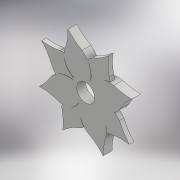
# Autodesk Inventor part: Hombro
Saved by Autodesk Inventor 2017 (Build 210142000, 142)
## iProperties
Created: 2018-06-14
Part Number: Hombro
Material: Generic
Document SubType Name: Modeling
Designer: Carolina Lema
Density: 1 g/cm^3
Appearance: Default
Author: Carolina Lema
Autodesk Inventor part; units mm, degrees
ref_plane "YZ Plane" through (0, 0, 0) normal (1, 0, 0) x (0, 1, 0)
ref_plane "XZ Plane" through (0, 0, 0) normal (0, 1, 0) x (-1, 0, 0)
ref_plane "XY Plane" through (0, 0, 0) normal (0, 0, 1) x (1, 0, 0)
sketch "Sketch1" plane through (0, 0, 0) normal (0, 1, 0) x (-1, 0, 0)
  circle A0 centre (0, 0) radius 3.1567
  arc A1 (0.8045, 7.8482) -> (-1.096, 2.9604) centre (3.8775, 3.84) ccw
  arc A2 (0.8045, 7.8482) -> (3.9995, 10.3658) centre (-5.1655, 18.7108) ccw
  arc A3 (3.9995, 10.3658) -> (4.6274, 6.3833) centre (14.1317, 9.9224) ccw
  arc A4 (2.723, 1.597) -> (4.6274, 6.3833) centre (0.993, 5.0574) ccw
  arc A5 (-2.811, -1.4364) -> (-4.581, -6.3031) centre (0.3797, -5.3521) ccw
  arc A6 (-3.9197, -10.3658) -> (-4.581, -6.3031) centre (-16.3145, -10.2983) ccw
  arc A7 (-0.7514, -7.7504) -> (-3.9197, -10.3658) centre (3.9871, -16.7173) ccw
  arc A8 (-0.7514, -7.7504) -> (1.0381, -2.9812) centre (-2.4622, -4.3882) ccw
  arc A9 (-4.581, 6.3031) -> (-3.9197, 10.3658) centre (-16.3145, 10.2983) ccw
  arc A10 (-3.9197, 10.3658) -> (-0.7514, 7.7504) centre (3.9871, 16.7173) ccw
  arc A11 (0.0827, -7.173) -> (0.8045, -7.8482) centre (3.8775, -3.84) ccw
  arc A12 (3.9995, -10.4433) -> (0.8045, -7.8482) centre (-5.3042, -18.6335) ccw
  arc A13 (4.6274, -6.3833) -> (3.9995, -10.4433) centre (14.1284, -9.9311) ccw
  arc A14 (4.6274, -6.3833) -> (4.8845, -4.8845) centre (1.1142, -5.0091) ccw
  arc A15 (-6.3833, -4.6274) -> (-4.6482, -4.8692) centre (-5.0091, -1.1142) ccw
  arc A16 (-1.4365, 2.8109) -> (-6.3031, 4.581) centre (-5.3521, -0.3794) ccw
  arc A17 (-7.7504, 0.7514) -> (-2.9812, -1.038) centre (-4.3883, 2.4621) ccw
  arc A18 (-6.3833, -4.6274) -> (-10.4433, -3.9995) centre (-9.9311, -14.1284) ccw
  arc A19 (-10.4433, -3.9995) -> (-7.8482, -0.8045) centre (-18.6335, 5.3042) ccw
  arc A20 (-7.7504, 0.7514) -> (-10.3658, 3.9197) centre (-16.7173, -3.9871) ccw
  arc A21 (-10.3658, 3.9197) -> (-6.3031, 4.581) centre (-10.2983, 16.3145) ccw
  arc A22 (-7.173, -0.0827) -> (-7.8482, -0.8045) centre (-3.84, -3.8775) ccw
  circle A23 centre (0, 0) radius 3.1567
  arc A24 (1.597, -2.723) -> (6.3833, -4.6274) centre (5.0091, -1.1142) ccw
  arc A25 (7.8482, -0.8045) -> (10.4433, -3.9995) centre (18.6335, 5.3042) ccw
  arc A26 (10.4433, -3.9995) -> (6.3833, -4.6274) centre (9.9311, -14.1284) ccw
  arc A27 (7.8482, -0.8045) -> (2.9604, 1.096) centre (3.84, -3.8775) ccw
  arc A28 (10.3658, 3.9197) -> (7.7544, 0.7514) centre (16.7241, -3.9816) ccw
  arc A29 (6.2595, 4.581) -> (10.3658, 3.9197) centre (10.2556, 16.3142) ccw
  arc A30 (-4.581, 6.3031) -> (-4.6176, 4.6176) centre (0.3794, 5.3521) ccw
  arc A31 (0.0827, 7.173) -> (-0.7514, 7.7504) centre (-2.4621, 4.3883) ccw
  arc A32 (6.2595, 4.581) -> (4.8322, 4.581) centre (5.5459, -0.4191) ccw
  arc A33 (7.173, -0.0827) -> (7.7544, 0.7514) centre (4.3971, 2.4718) ccw
  point P0 (0, 0)
  constraints: 82 point on circle, 34 centre point
extrude "Extrusion1" add sketch "Sketch1" along normal blind 2 contours A0 | A0 A27 A25 A26 A24 | A0 A1 A2 A3 A4 | A8 A7 A6 A5 A0 | A0 A17 A20 A21 A16
sketch "Sketch2" plane through (0, 0, 0) normal (0, -1, 0) x (1, 0, 0)
  arc A0 (-6.3002, -4.5761) -> (-10.3587, -3.9384) centre (-9.8712, -14.0685) ccw
  arc A1 (-10.3587, -3.9384) -> (-7.7558, -0.7497) centre (-18.5261, 5.3853) ccw
  arc A2 (-7.6963, 1.7106) -> (-6.727, 0.2513) centre (-4.1552, 3.0112) ccw
  arc A3 (-7.6963, 1.7106) -> (-9.9181, 5.1662) centre (-17.1611, -1.9329) ccw
  arc A4 (1.6813, 7.6084) -> (0.3953, 6.5184) centre (4.2581, 3.2645) ccw
  arc A5 (5.4246, 4.6938) -> (5.3039, 5.7011) centre (1.6527, 4.7526) ccw
  arc A6 (5.1612, 9.8069) -> (5.3039, 5.7011) centre (15.1582, 8.099) ccw
  arc A7 (1.6813, 7.6084) -> (5.1612, 9.8069) centre (-3.1073, 19.0411) ccw
  circle A8 centre (0, 0) radius 3.1567
  arc A9 (-2.939, 1.152) -> (-7.7558, -0.7497) centre (-3.7548, -3.8328) ccw
  arc A10 (-3.9384, 10.3587) -> (-0.7497, 7.7558) centre (5.3853, 18.5261) ccw
  arc A11 (1.1518, 2.9391) -> (-0.7497, 7.7558) centre (-3.8325, 3.7551) ccw
  arc A12 (-4.5761, 6.3002) -> (-3.9384, 10.3587) centre (-14.0685, 9.8712) ccw
  arc A13 (-4.8177, 5.3149) -> (-5.8057, 5.3418) centre (-5.4487, 0.3038) ccw
  arc A14 (-9.9181, 5.1662) -> (-5.8057, 5.3418) centre (-8.3835, 17.4659) ccw
  arc A15 (-4.5761, 6.3002) -> (-2.7536, 1.5435) centre (-1.0663, 4.9175) ccw
  circle A16 centre (0, 0) radius 3.1567
  arc A17 (7.5795, -1.6487) -> (9.8069, -5.1612) centre (19.0125, 3.1391) ccw
  arc A18 (9.8069, -5.1612) -> (5.7037, -5.3068) centre (8.1076, -15.1596) ccw
  arc A19 (7.5795, -1.6487) -> (6.6332, -0.5802) centre (3.3633, -4.4295) ccw
  arc A20 (10.4117, 3.8786) -> (7.8466, 0.7681) centre (16.7974, -4.0005) ccw
  arc A21 (4.6938, -5.4246) -> (5.7037, -5.3068) centre (4.7657, -1.6529) ccw
  arc A22 (6.4086, 4.6012) -> (10.4117, 3.8786) centre (10.5823, 16.2725) ccw
  arc A23 (3.0009, -0.9796) -> (7.8466, 0.7681) centre (4.4443, 2.6098) ccw
  arc A24 (6.4086, 4.6012) -> (1.4895, 2.7832) centre (5.4455, -0.3568) ccw
  arc A25 (4.6012, -6.4086) -> (2.7832, -1.4895) centre (-0.3568, -5.4455) ccw
  arc A26 (-1.7106, -7.6963) -> (-5.1662, -9.9181) centre (1.9329, -17.1611) ccw
  arc A27 (-1.7106, -7.6963) -> (-0.4181, -6.895) centre (-3.0112, -4.1552) ccw
  arc A28 (-5.1662, -9.9181) -> (-5.3418, -5.8057) centre (-17.4659, -8.3835) ccw
  arc A29 (3.9299, -10.4697) -> (0.7681, -7.8466) centre (-3.9923, -16.8018) ccw
  arc A30 (-5.3149, -4.8177) -> (-5.3418, -5.8057) centre (-0.3038, -5.4487) ccw
  arc A31 (4.6012, -6.4086) -> (3.9299, -10.4697) centre (16.3249, -10.4325) ccw
  arc A32 (-0.9796, -3.0009) -> (0.7681, -7.8466) centre (2.487, -4.4886) ccw
  arc A33 (-6.3002, -4.5761) -> (-1.5435, -2.7537) centre (-4.9175, -1.0662) ccw
  point P0 (0, 0)
  point P1 (0, 0)
  constraints: 82 point on circle, 34 centre point
extrude "Extrusion2" add sketch "Sketch2" against normal blind 1 contours A33 A8 A32 A27 A26 A28 A30 | A8 | A2 A3 A14 A13 A15 A8 A9 | A8 A23 A19 A17 A18 A21 A25 | A11 A4 A7 A6 A5 A24 A8
sketch "Sketch3" plane through (0, 2, 0) normal (0, 1, 0) x (1, 0, 0)
  circle A0 centre (0, 0) radius 2
  dimension "d4" = 4
  constraints: 1 centre point, 1 coincident
  measures "d4" diameter of A0
extrude "Extrusion3" cut sketch "Sketch3" against normal blind 2
body "Solid1"
